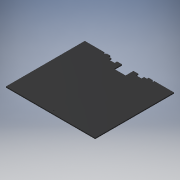
# Autodesk Inventor part: ElectronicsTopPanel
Saved by Autodesk Inventor 2016 (Build 200138000, 138)
## iProperties
Category: Panel
Created: 2015-01-14
Part Number: ElectronicsTopPanel
Material: ABS Plastic
Document SubType Name: Modeling
Designer: Jack
Density: 1.06 g/cm^3
Appearance: Smooth - Dark Gray
Mass: 810.36 g
Surface Area: 3294.73 cm^2
Volume: 764.49 cm^3
Author: Jack
Title: Electronics Top Panel
Autodesk Inventor part; units mm, degrees
ref_plane "YZ Plane" through (0, 0, 0) normal (1, 0, 0) x (0, 1, 0)
ref_plane "XZ Plane" through (0, 0, 0) normal (0, 1, 0) x (-1, 0, 0)
ref_plane "XY Plane" through (0, 0, 0) normal (0, 0, 1) x (1, 0, 0)
sketch "Sketch1" plane through (0, 0, 0) normal (0, 0, 1) x (1, 0, 0)
  line L0 (0, 0) -> (430, 0)
  line L1 (430, 0) -> (430, 380)
  line L2 (430, 380) -> (0, 380)
  line L3 (0, 380) -> (0, 0)
  dimension "d0" = 430
  dimension "d1" = 380
  constraints: 8 end point, 2 parallel, 1 horizontal, 1 perpendicular
  measures "d0" distance of L2.end L1.end
  measures "d1" distance of L1.end L0.end
extrude "Extrusion1" add sketch "Sketch1" along normal blind 4.7625
sketch "Sketch2" plane through (0, 0, 4.7625) normal (0, 0, 1) x (1, 0, 0)
  line L0 (0, 0) -> (430, 0) projected
  line L1 (430, 0) -> (430, 380) projected
  point P0 (215, 16)
  dimension "d8" = 215
  dimension "d33" = 16
  measures "d8" distance from line of L1 point (215, 16)
  measures "d33" distance from line of L0 point (215, 16)
hole "Hole1" at (215, 16, 4.7625) direction (0, 0, -1) diameter 3 end through all
sketch "Sketch4" plane through (0, 0, 4.7625) normal (0, 0, 1) x (1, 0, 0)
  line L0 (430, 380) -> (0, 380) projected
  line L1 (122.5, 380) -> (122.5, 372)
  line L2 (122.5, 372) -> (136.5, 372)
  line L3 (136.5, 372) -> (136.5, 360)
  line L4 (136.5, 360) -> (163.5, 360)
  line L5 (163.5, 360) -> (163.5, 372)
  line L6 (163.5, 372) -> (187.5, 372)
  line L7 (187.5, 372) -> (187.5, 334)
  line L8 (187.5, 334) -> (242.5, 334)
  line L9 (242.5, 334) -> (242.5, 372)
  line L10 (242.5, 372) -> (266.5, 372)
  line L11 (266.5, 372) -> (266.5, 360)
  line L12 (266.5, 360) -> (293.5, 360)
  line L13 (293.5, 360) -> (293.5, 372)
  line L14 (293.5, 372) -> (307.5, 372)
  line L15 (307.5, 372) -> (307.5, 380)
  point P0 (215, 380)
  point P1 (215, 334)
  dimension "d20" = 14
  dimension "d21" = 8
  dimension "d22" = 12
  dimension "d23" = 14
  dimension "d24" = 27
  dimension "d25" = 27
  dimension "d26" = 24
  dimension "d27" = 38
  dimension "d28" = 24
  dimension "d31" = 55
  constraints: 30 end point, 11 perpendicular, 8 point on line, 2 midpoint, 1 horizontal alignment, 1 vertical, 1 vertical alignment
  measures "d20" distance between parallel lines of L15 L13
  measures "d21" distance between parallel lines of L0 L14
  measures "d22" distance between parallel lines of L6 L4
  measures "d23" distance of L1.end L2.end
  measures "d24" distance of L3.end L4.end
  measures "d25" distance of L11.end L12.end
  measures "d26" distance between parallel lines of L11 L9
  measures "d27" distance between parallel lines of L10 L8
  measures "d28" distance between parallel lines of L5 L7
  measures "d31" distance of L7.end L8.end
extrude "Extrusion2" cut sketch "Sketch4" against normal up to next
sketch "Sketch5" plane through (0, 0, 4.7625) normal (0, 0, 1) x (1, 0, 0)
  line L0 (122.5, 380) -> (0, 380) projected
  line L1 (0, 380) -> (0, 0) projected
  line L2 (430, 0) -> (430, 380) projected
  line L3 (430, 380) -> (307.5, 380) projected
  line L4 (94, 380) -> (94, 374)
  line L5 (94, 374) -> (102, 374)
  line L6 (102, 374) -> (102, 380)
  line L7 (327, 380) -> (327, 374)
  line L8 (327, 374) -> (335, 374)
  line L9 (335, 374) -> (335, 380)
  dimension "d36" = 8
  dimension "d37" = 94
  dimension "d38" = 6
  dimension "d39" = 95
  constraints: 12 end point, 4 perpendicular, 4 point on line, 2 vertical, 1 collinear, 1 horizontal alignment
  measures "d36" distance of L4.end L5.end
  measures "d37" distance between parallel lines of L1 L4
  measures "d38" distance of L5.end L6.end
  measures "d39" distance between parallel lines of L2 L9
extrude "Extrusion3" cut sketch "Sketch5" against normal up to next
sketch "Sketch6" plane through (0, 0, 4.7625) normal (0, 0, 1) x (1, 0, 0)
  line L0 (102, 380) -> (106, 380)
  line L1 (106, 380) -> (106, 377)
  line L2 (106, 377) -> (102, 377)
  line L3 (102, 377) -> (102, 380)
  dimension "d42" = 4
  dimension "d43" = 3
  constraints: 8 end point, 2 parallel, 1 horizontal, 1 perpendicular
  measures "d42" distance of L1.end L2.end
  measures "d43" distance of L0.end L1.end
extrude "Extrusion4" cut sketch "Sketch6" against normal up to next
body "Solid1"
